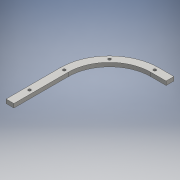
# Autodesk Inventor part: side_walls
Saved by Autodesk Inventor 2016 (Build 200138000, 138)
## iProperties
Created: 2015-09-09
Part Number: side_walls
Material: Generic
Document SubType Name: Modeling
Designer: oscar
Density: 1 g/cm^3
Appearance: Default
Author: oscar
Autodesk Inventor part; units mm, degrees
ref_plane "YZ Plane" through (0, 0, 0) normal (1, 0, 0) x (0, 1, 0)
ref_plane "XZ Plane" through (0, 0, 0) normal (0, 1, 0) x (-1, 0, 0)
ref_plane "XY Plane" through (0, 0, 0) normal (0, 0, 1) x (1, 0, 0)
sketch "Sketch1" plane through (0, 0, 0) normal (0, 0, 1) x (1, 0, 0)
  arc A0 (763.7742, 1811.2181) -> (637.7742, 1685.2181) centre (763.7742, 1685.2181) ccw
  arc A1 (763.7742, 1791.2181) -> (657.7742, 1685.2181) centre (763.7742, 1685.2181) ccw
  line L0 (637.7742, 1546.2181) -> (657.7742, 1546.2181)
  circle A2 centre (763.7742, 1801.2181) radius 3.5
  circle A3 centre (647.7742, 1596.2181) radius 3.5
  circle A4 centre (647.7742, 1685.2181) radius 3.5
  line L1 (802.7742, 1811.2181) -> (802.7742, 1791.2181)
  circle A5 centre (681.7499, 1767.2425) radius 3.5
  line L2 (637.7742, 1685.2181) -> (637.7742, 1546.2181)
  line L3 (657.7742, 1546.2181) -> (657.7742, 1685.2181)
  line L4 (763.7742, 1791.2181) -> (802.7742, 1791.2181)
  line L5 (802.7742, 1811.2181) -> (763.7742, 1811.2181)
  point P0 (0, 0)
  constraints: 12 end point, 6 centre point, 4 point on circle, 2 parallel, 1 perpendicular, 1 vertical
extrude "Extrusion1" add sketch "Sketch1" along normal blind 10
body "Solid1"
